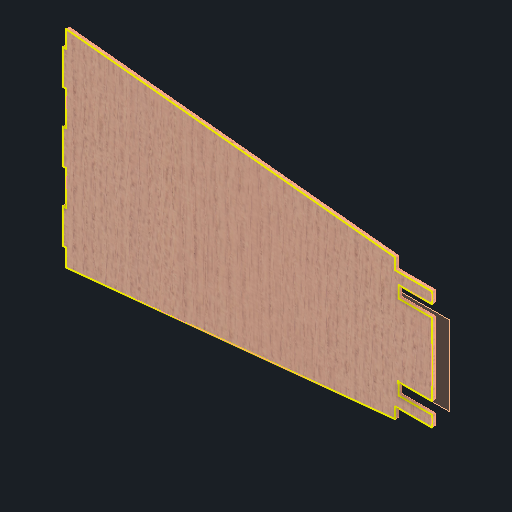
# Autodesk Inventor part: Stand 1
Saved by Autodesk Inventor 2025.2 (Build 292293000, 293)
## iProperties
Created: 2024-11-19
Part Number: Stand 1
Material: Wood (Oak)
Document SubType Name: Modeling
Designer: JL
Density: 0.76 g/cm^3
Appearance: White Oak - Natural Medium Gloss
Author: JL
Autodesk Inventor part; units mm, degrees
ref_plane "YZ Plane" through (0, 0, 0) normal (1, 0, 0) x (0, 1, 0)
ref_plane "XZ Plane" through (0, 0, 0) normal (0, 1, 0) x (-1, 0, 0)
ref_plane "XY Plane" through (0, 0, 0) normal (0, 0, 1) x (1, 0, 0)
ref_plane "Work Plane1" through (0, 0, 0) normal (0, 0, 1) x (1, 0, 0)
sketch "Sketch1" plane through (0, 0, 0) normal (0, 0, 1) x (1, 0, 0)
  line L0 (0, 75.8) -> (40.7, 75.8) projected
  line L1 (40.7, 65.2) -> (40.7, 75.8) construction
  line L2 (40.7, 65.2) -> (0, 65.2) projected
  line L3 (0, 65.2) -> (0, 75.8) projected
  line L4 (0, 0) -> (0, 65.2) construction
  line L5 (40.7, 0) -> (0, 0) projected
  line L6 (40.7, 0) -> (40.7, 65.2) construction
  line L7 (0, 65.2) -> (40.7, 65.2) projected
  line L8 (0, -10.6) -> (40.7, -10.6) projected
  line L9 (0, 0) -> (0, -10.6)
  line L10 (40.7, -10.6) -> (40.7, 0) construction
  line L11 (40.7, 32.6) -> (0, 32.6) construction
  line L12 (0, 32.6) -> (-300, 32.6) construction
  line L13 (30, 75.8) -> (30, 85.8)
  line L14 (-300, 125.8) -> (-300, 32.6)
  line L15 (-300, -60.6) -> (-300, 32.6)
  line L16 (30, 0) -> (30, 65.2)
  line L17 (-3, 85.8) -> (-3, 95.8)
  line L18 (30, 85.8) -> (-3, 85.8)
  line L19 (-3, 95.8) -> (-300, 125.8)
  line L20 (30, -10.6) -> (30, -20.6)
  line L21 (-3, -20.6) -> (-3, -30.6)
  line L22 (30, -20.6) -> (-3, -20.6)
  line L23 (-3, -30.6) -> (-300, -60.6)
  line L24 (-300, 110.2667) -> (-303, 110.2667)
  line L25 (-303, 110.2667) -> (-303, 79.2)
  line L26 (-303, 79.2) -> (-300, 79.2)
  line L27 (-300, 48.1333) -> (-303, 48.1333)
  line L28 (-303, 48.1333) -> (-303, 32.6)
  line L29 (-303, 32.6) -> (-300, 32.6) construction
  line L30 (-303, 79.2) -> (-303, 48.1333) construction
  line L31 (-303, 110.2667) -> (-303, 125.8) construction
  line L32 (-303, 125.8) -> (-300, 125.8) construction
  line L33 (-301.5, 110.2667) -> (-301.5, 94.7333) construction
  line L34 (-301.5, 94.7333) -> (-303, 94.7333) construction
  line L35 (-300, -45.0667) -> (-303, -45.0667)
  line L36 (-303, -45.0667) -> (-303, -14)
  line L37 (-303, -14) -> (-300, -14)
  line L38 (-300, 17.0667) -> (-303, 17.0667)
  line L39 (-303, 17.0667) -> (-303, 32.6)
  line L40 (-3, 75.8) -> (-3, 85.8) projected
  dimension "d0" = 300
  dimension "d1" = 10
  dimension "d2" = 50
  dimension "d3" = 30
  dimension "d6" = 10
  dimension "d10" = 3
  constraints: 62 end point, 11 symmetric about line, 10 perpendicular, 10 point on line, 5 midpoint, 3 collinear, 3 equal length, 3 vertical, 2 horizontal, 1 parallel
  measures "d0" distance of L11.end L12.end
  measures "d1" distance of L13.start L13.end
  measures "d2" vertical distance of L14.start L0.start
  measures "d3" distance from line of L0.start L13
  measures "d6" distance of L17.start L17.end
  measures "d10" distance of L24.start L24.end
extrude "Extrusion1" add sketch "Sketch1" along normal blind 3
sketch "Sketch3" plane through (0, 0, 3) normal (0, 0, 1) x (1, 0, 0)
  line L0 (0, 75.8) -> (30, 75.8) projected
  line L1 (30, 75.8) -> (30, 85.8) projected
  line L2 (30, 85.8) -> (-3, 85.8) projected
  line L3 (-3, 85.8) -> (-3, 95.8) projected
  line L4 (-3, 95.8) -> (-300, 125.8) projected
  line L5 (-300, 125.8) -> (-300, 110.2667) projected
  line L6 (-300, 110.2667) -> (-303, 110.2667) projected
  line L7 (-303, 110.2667) -> (-303, 79.2) projected
  line L8 (-303, 79.2) -> (-300, 79.2) projected
  line L9 (-300, 79.2) -> (-300, 48.1333) projected
  line L10 (-300, 48.1333) -> (-303, 48.1333) projected
  line L11 (-303, 48.1333) -> (-303, 17.0667) projected
  line L12 (-303, 17.0667) -> (-300, 17.0667) projected
  line L13 (-300, 17.0667) -> (-300, -14) projected
  line L14 (-300, -14) -> (-303, -14) projected
  line L15 (-303, -14) -> (-303, -45.0667) projected
  line L16 (-303, -45.0667) -> (-300, -45.0667) projected
  line L17 (-300, -45.0667) -> (-300, -60.6) projected
  line L18 (-300, -60.6) -> (-3, -30.6) projected
  line L19 (-3, -30.6) -> (-3, -20.6) projected
  line L20 (-3, -20.6) -> (30, -20.6) projected
  line L21 (30, -20.6) -> (30, -10.6) projected
  line L22 (30, -10.6) -> (0, -10.6) projected
  line L23 (0, -10.6) -> (0, 0) projected
  line L24 (0, 0) -> (30, 0) projected
  line L25 (30, 0) -> (30, 65.2) projected
  line L26 (30, 65.2) -> (0, 65.2) projected
  line L27 (0, 65.2) -> (0, 75.8) projected
body "Solid1"
